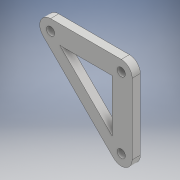
# Autodesk Inventor part: barra_tri
Saved by Autodesk Inventor 2018 (Build 220112000, 112)
## iProperties
Created: 2018-05-25
Part Number: barra_tri
Material: Generic
Document SubType Name: Modeling
Designer: vigus
Density: 1 g/cm^3
Appearance: Default
Author: vigus
Autodesk Inventor part; units mm, degrees
ref_plane "YZ Plane" through (0, 0, 0) normal (1, 0, 0) x (0, 1, 0)
ref_plane "XZ Plane" through (0, 0, 0) normal (0, 1, 0) x (-1, 0, 0)
ref_plane "XY Plane" through (0, 0, 0) normal (0, 0, 1) x (1, 0, 0)
sketch "Sketch2" plane through (0, 0, 0) normal (0, 1, 0) x (-1, 0, 0)
  circle A0 centre (0, 0) radius 1.5
  circle A1 centre (0, 0) radius 4
  line L0 (0, 0) -> (26, 0)
  circle A2 centre (26, 0) radius 1.5
  circle A3 centre (26, 0) radius 4
  line L1 (0, 0) -> (0, -26)
  circle A4 centre (0, -26) radius 1.5
  circle A5 centre (0, -26) radius 4
  line L2 (-4, 0) -> (-4, -26)
  line L3 (26, 4) -> (0, 4)
  line L4 (28.8284, -2.8284) -> (2.8284, -28.8284)
  line L5 (17.8965, -2.8284) -> (3.3271, -2.8284)
  line L6 (3.3271, -2.8284) -> (3.3271, -22.0752)
  line L7 (3.3271, -22.0752) -> (22.5739, -2.8284)
  line L8 (22.5739, -2.8284) -> (17.3203, -2.8284)
  dimension "d1" = 3
  dimension "d2" = 8
  dimension "d3" = 26
  dimension "d4" = 3
  dimension "d5" = 8
  dimension "d6" = 26
  dimension "d7" = 3
  dimension "d8" = 8
  constraints: 18 end point, 6 centre point, 6 coincident, 6 point on circle, 4 tangent, 3 horizontal, 2 point on line, 2 vertical, 1 perpendicular
  measures "d1" diameter of A0
  measures "d2" diameter of A1
  measures "d3" distance of L0.start L0.end
  measures "d4" diameter of A2
  measures "d5" diameter of A3
  measures "d6" distance of L0.start L1.end
  measures "d7" diameter of A4
  measures "d8" diameter of A5
extrude "Extrusion1" add sketch "Sketch2" along normal blind 3 contours L0 A1 L1 A0 | A0 L1 A1 L0 | L0 A3 L4 A5 L1 A1 | A1 L3 A3 L0 | L1 A5 L2 A1 | A3 | A5
body "Solid1"
